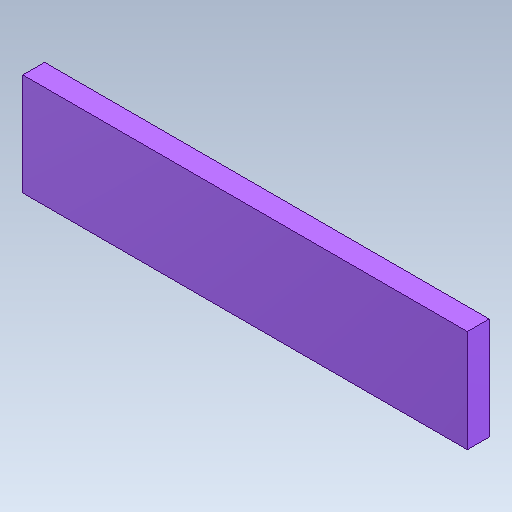
# Autodesk Inventor part: OPA549T
Saved by Autodesk Inventor 2021 (Build 250183000, 183)
## iProperties
Created: 2020-11-18
Part Number: OPA549T
Material: Generic
Document SubType Name: Modeling
Designer: Admin
Density: 1 g/cm^3
Appearance: KV11, OPA549T
Author: Admin
Autodesk Inventor part; units mm, degrees
ref_plane "YZ Plane" through (0, 0, 0) normal (1, 0, 0) x (0, 1, 0)
ref_plane "XZ Plane" through (0, 0, 0) normal (0, 1, 0) x (-1, 0, 0)
ref_plane "XY Plane" through (0, 0, 0) normal (0, 0, 1) x (1, 0, 0)
sketch "KV11, OPA549T_61" plane through (0, 0, 0) normal (0, 0, 1) x (1, 0, 0)
  line L0 (-18.7198, 1.778) -> (1.7018, 1.778)
  line L1 (1.7018, 1.778) -> (1.7018, -2.921)
  line L2 (1.7018, -2.921) -> (-18.7198, -2.921)
  line L3 (-18.7198, -2.921) -> (-18.7198, 1.778)
  constraints: 8 end point
extrude "Extrusion1" add sketch "KV11, OPA549T_61" along normal blind 1
body "Solid1"
